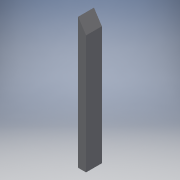
# Autodesk Inventor part: ramp angle 1
Saved by Autodesk Inventor 2018.2 (Build 222227000, 227)
## iProperties
Created: 2018-01-29
Part Number: ramp angle 1
Material: Generic
Document SubType Name: Modeling
Designer: Orangeracer
Density: 1 g/cm^3
Appearance: Default
Author: Orangeracer
Autodesk Inventor part; units mm, degrees
ref_plane "YZ Plane" through (0, 0, 0) normal (1, 0, 0) x (0, 1, 0)
ref_plane "XZ Plane" through (0, 0, 0) normal (0, 1, 0) x (-1, 0, 0)
ref_plane "XY Plane" through (0, 0, 0) normal (0, 0, 1) x (1, 0, 0)
sketch "Sketch1" plane through (0, 0, 0) normal (0, 0, 1) x (1, 0, 0)
  line L0 (0, 0) -> (-25.4, 0)
  line L1 (-25.4, 0) -> (-25.4, -381)
  line L2 (-25.4, -381) -> (0, -381)
  line L3 (0, -381) -> (0, 0)
  line L4 (0, 0) -> (-25.4, 0)
  line L5 (-25.4, 0) -> (-25.4, 12.7)
  line L6 (0, 0) -> (-25.4, 12.7)
  dimension "d0" = 25.4
  dimension "d1" = 381
  dimension "d3" = 12.7
  dimension "d7" = 25.4
  constraints: 14 end point, 2 horizontal, 2 parallel, 2 perpendicular
  measures "d0" distance of L2.end L1.end
  measures "d1" distance of L1.end L0.end
  measures "d3" distance of L4.end L5.end
  measures "d7" distance of L0.start L4.end
extrude "Extrusion1" add sketch "Sketch1" along normal blind 50.8
body "Solid1"
